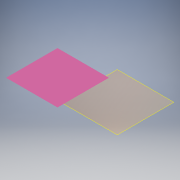
# Autodesk Inventor part: Sitzfläche
Saved by Autodesk Inventor 2018.3 (Build 223284000, 284)
## iProperties
Created: 2019-09-20
Part Number: Sitzfläche
Material: Generisch
Document SubType Name: Modeling
Designer: Lolob
Density: 1 g/cm^3
Appearance: Vorgabe
Author: Lolob
Title: SitzFläche
Autodesk Inventor part; units mm, degrees
ref_plane "YZ Plane" through (0, 0, 0) normal (1, 0, 0) x (0, 1, 0)
ref_plane "XZ Plane" through (0, 0, 0) normal (0, 1, 0) x (-1, 0, 0)
ref_plane "XY Plane" through (0, 0, 0) normal (0, 0, 1) x (1, 0, 0)
ref_plane "Arbeitsebene1" through (-858.9244, 0, 0) normal (0, 0, 1) x (1, 0, 0)
sketch "Skizze2" plane through (-858.9244, 0, 0) normal (0, 0, 1) x (1, 0, 0)
  line L0 (-0.0619, 347.3197) -> (439.9381, 347.3197)
  line L1 (439.9381, 347.3197) -> (439.9381, -92.6803)
  line L2 (439.9381, -92.6803) -> (-0.0619, -92.6803)
  line L3 (-0.0619, -92.6803) -> (-0.0619, 347.3197)
  point P0 (858.9244, 0)
  dimension "d5" = 440
  dimension "d6" = 440
  constraints: 8 end point, 2 parallel, 1 horizontal, 1 perpendicular
  measures "d5" distance of L0.start L0.end
  measures "d6" distance of L0.end L1.end
extrude "Extrusion2" add sketch "Skizze2" along normal blind 18
chamfer "Fase2" distance 18 angle 45 4 edges at (-638.9863, -92.6803, 0) (-418.9863, 127.3197, 0) (-858.9863, 127.3197, 0) (-638.9863, 347.3197, 0)
sketch "Skizze3" plane through (-858.9244, 0, 0) normal (0, 0, -1) x (-1, 0, 0)
  line L0 (-41.9381, -54.6803) -> (-83.9381, -54.6803)
  line L1 (-87.9381, -50.6803) -> (-87.9381, 31.3197)
  line L2 (-83.9381, 35.3197) -> (-41.9381, 35.3197)
  line L3 (-37.9381, 31.3197) -> (-37.9381, -50.6803)
  line L4 (-17.9381, -74.6803) -> (-421.9381, -74.6803) projected
  line L5 (-17.9381, 329.3197) -> (-17.9381, -74.6803) projected
  arc A0 (-41.9381, -54.6803) -> (-37.9381, -50.6803) centre (-41.9381, -50.6803) ccw
  arc A1 (-87.9381, -50.6803) -> (-83.9381, -54.6803) centre (-83.9381, -50.6803) ccw
  arc A2 (-83.9381, 35.3197) -> (-87.9381, 31.3197) centre (-83.9381, 31.3197) ccw
  arc A3 (-37.9381, 31.3197) -> (-41.9381, 35.3197) centre (-41.9381, 31.3197) ccw
  point P0 (-858.9244, 0)
  point P1 (-87.9381, 35.3197)
  point P2 (-87.9381, -54.6803)
  point P3 (-37.9381, 35.3197)
  dimension "d12" = 50
  dimension "d13" = 90
  dimension "d14" = 20
  dimension "d15" = 20
  dimension "d16" = 4
  constraints: 8 end point, 8 point on circle, 8 tangent, 6 point on line, 4 centre point, 3 equal radius, 2 parallel, 1 horizontal, 1 perpendicular
  measures "d12" distance of point (-87.938, 35.32) point (-37.938, 35.32)
  measures "d13" distance of point (-87.938, -54.68) point (-87.938, 35.32)
  measures "d14" distance between parallel lines of L4 L0
  measures "d15" distance between parallel lines of L5 L3
  measures "d16" radius of A0
extrude "Extrusion3" cut sketch "Skizze3" against normal blind 15
